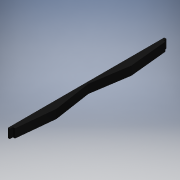
# Autodesk Inventor part: long_insert_CPY
Saved by Autodesk Inventor 2017 (Build 210142000, 142)
## iProperties
Created: 2018-01-14
Part Number: long_insert_CPY
Material: Generic
Document SubType Name: Modeling
Designer: Mitch
Density: 1 g/cm^3
Appearance: Glossy - Black
Author: Mitch
Autodesk Inventor part; units mm, degrees
ref_plane "YZ Plane" through (0, 0, 0) normal (1, 0, 0) x (0, 1, 0)
ref_plane "XZ Plane" through (0, 0, 0) normal (0, 1, 0) x (-1, 0, 0)
ref_plane "XY Plane" through (0, 0, 0) normal (0, 0, 1) x (1, 0, 0)
sketch "Sketch1" plane through (0, 0, 0) normal (0, 1, 0) x (-1, 0, 0)
  line L0 (0, 0) -> (0, -125.2474)
  line L1 (0, -125.2474) -> (-3.4036, -125.2474)
  line L2 (0, 0) -> (-3.4036, 0)
  line L3 (-3.4036, 0) -> (-6.5786, -31.3753)
  line L4 (-6.5786, -31.3753) -> (-1.778, -62.7507)
  line L5 (-1.778, -62.7507) -> (-6.5786, -93.8721)
  line L6 (-6.5786, -93.8721) -> (-3.4036, -125.2474)
  dimension "d0" = 125.2474
  dimension "d1" = 3.4036
  dimension "d2" = 3.4036
  dimension "d3" = 31.3754
  dimension "d4" = 62.7507
  dimension "d5" = 31.3754
  dimension "d6" = 3.175
  dimension "d7" = 3.175
  constraints: 14 end point, 2 horizontal, 1 vertical
  measures "d0" distance of L0.start L0.end
  measures "d1" distance of L0.end L1.end
  measures "d2" distance of L0.start L2.end
  measures "d3" distance from line of L3.end L2
  measures "d4" distance from line of L4.end L2
  measures "d5" distance from line of L5.end L1
  measures "d6" horizontal distance of L3.end L2.end
  measures "d7" horizontal distance of L5.end L1.end
extrude "Extrusion1" add sketch "Sketch1" along normal blind 7.3025
sketch "Sketch2" plane through (0, 0, 0) normal (0, 0, 1) x (1, 0, 0)
  line L0 (0, 0) -> (0, 7.3025) projected
  line L1 (3.4036, 0) -> (0, 0) projected
  line L2 (0, 7.3025) -> (1.651, 7.3025)
  line L3 (1.651, 7.3025) -> (1.651, 0)
  line L4 (1.651, 0) -> (0, 0)
  line L5 (0, 0) -> (0, 7.3025)
  dimension "d10" = 1.651
  constraints: 8 end point, 2 parallel, 1 horizontal, 1 perpendicular, 1 point on line
  measures "d10" distance of L3.end L4.end
sketch "Sketch3" plane through (3.4036, 0, -125.2474) normal (0, 0, -1) x (-1, 0, 0)
  line L0 (0, 0) -> (3.4036, 0) projected
  line L1 (3.4036, 7.3025) -> (1.7526, 7.3025)
  line L2 (1.7526, 7.3025) -> (1.7526, 0)
  line L3 (1.7526, 0) -> (3.4036, 0)
  line L4 (3.4036, 0) -> (3.4036, 7.3025)
  dimension "d11" = 1.651
  constraints: 8 end point, 2 parallel, 1 horizontal, 1 perpendicular, 1 point on line
  measures "d11" distance of L3.end L2.end
extrude "Extrusion2" add sketch "Sketch2" along normal blind 2.5654
extrude "Extrusion3" add sketch "Sketch3" along normal blind 2.5654
body "Solid1"
